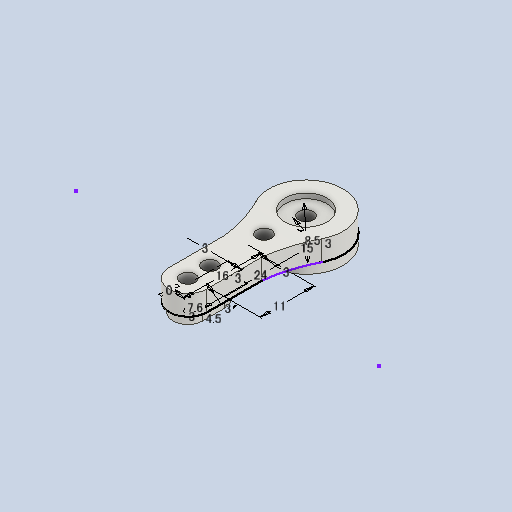
# Autodesk Inventor part: ServoMotor_Hone2
Saved by Autodesk Inventor 2022 (Build 260153000, 153)
## iProperties
Created: 2024-09-23
Part Number: ServoMotor_Hone2
Material: 鋼、高強度、低合金
Document SubType Name: Modeling
Designer: acbaf
Density: 7.85 g/cm^3
Appearance: 鋼
Author: acbaf
Autodesk Inventor part; units mm, degrees
ref_plane "YZ Plane" through (0, 0, 0) normal (1, 0, 0) x (0, 1, 0)
ref_plane "XZ Plane" through (0, 0, 0) normal (0, 1, 0) x (-1, 0, 0)
ref_plane "XY Plane" through (0, 0, 0) normal (0, 0, 1) x (1, 0, 0)
sketch "スケッチ1" plane through (0, 0, 0) normal (0, 1, 0) x (-1, 0, 0)
  circle A0 centre (0, 0) radius 7.5
  circle A1 centre (0, 0) radius 4.25
  circle A2 centre (0, 0) radius 1.5
  line L0 (0, 0) -> (0, 24)
  circle A3 centre (0, 24) radius 3.8
  line L1 (3.8, 24) -> (3.8, 12.8013)
  line L2 (-3.8, 24) -> (-3.8, 12.8013)
  circle A4 centre (0, 24) radius 1.5
  circle A5 centre (0, 19.5) radius 1.5
  circle A6 centre (0, 8.5) radius 1.5
  arc A7 (3.8, 12.8013) -> (6.6601, 3.4487) centre (30.7804, 15.9384) ccw
  arc A8 (-6.6601, 3.4487) -> (-3.8, 12.8013) centre (-30.7804, 15.9384) ccw
  line L3 (-3, 19.487) -> (3, 19.487)
  line L4 (3, 19.487) -> (3, 24.0195)
  line L5 (3, 24.0195) -> (-3, 24.0195)
  line L6 (-3, 24.0195) -> (-3, 19.487)
  circle A9 centre (0, 19.487) radius 3
  circle A10 centre (0, 24.0195) radius 3
  point P0 (3.8, 8)
  point P1 (-3.8, 8)
  point P2 (-6.6601, 3.4487)
  point P3 (3.8, 24)
  point P4 (-1.0476, 7.4265)
  point P5 (1.0476, 7.4265)
  dimension "d0" = 15
  dimension "d1" = 8.5
  dimension "d2" = 3
  dimension "d3" = 24
  dimension "d4" = 7.6
  dimension "d5" = 16
  dimension "d6" = 0
  dimension "d7" = 3
  dimension "d8" = 3
  dimension "d9" = 4.5
  dimension "d10" = 3
  dimension "d11" = 11
  dimension "d14" = 3
  dimension "d15" = 3
  constraints: 14 end point, 9 centre point, 5 coincident, 5 symmetric about line, 4 point on circle, 2 midpoint, 2 parallel, 2 point on line, 2 tangent, 2 vertical, 1 horizontal, 1 perpendicular, 8 other
  measures "d1" diameter of A1
  measures "d2" diameter of A2
  measures "d3" distance of L0.start L0.end
  measures "d4" diameter of A3
  measures "d5" distance of L1.start point (3.8, 8)
  measures "d6" vertical distance of L1.start A3.centre
  measures "d7" diameter of A4
  measures "d8" diameter of A5
  measures "d9" distance of A5.centre L0.end
  measures "d10" diameter of A6
  measures "d11" distance of A6.centre A5.centre
  measures "d14" distance between parallel lines of L0 L6
  measures "d15" distance between parallel lines of L4 L0
extrude "押し出し1" add sketch "スケッチ1" along normal blind 4 contours A0 A6 | A0 A6 L0 A9 L4 A3 L1 A7 | A8 L2 A3 L6 A9 L0 A6 A0 | A3 L4 A10 L6 | L4 A9 A3 | A3 A9 A10 L4 | A9 L3 A5 L0 | L0 A5 L3 A9 | L6 A10 A9 A3 | A3 A9 L6 | A9 L3 A5 A3 | A3 A5 L0 A10 A9 | A10 A9 L0 A4 L5 | L5 A4 A10 | A9 A3 A5 L3 | A9 A10 L0 A5 A3 | L5 A4 L0 A9 A10 | A10 L0 A9 | A9 L0 A10
extrude "押し出し2" add sketch "スケッチ1" against normal blind 2 contours L4 A9 A3 | A3 A9 A10 L4 | A9 L3 A5 L0 | L0 A5 L3 A9 | L6 A10 A9 A3 | A3 A9 L6 | A9 L3 A5 A3 | A3 A5 L0 A10 A9 | A10 A9 L0 A4 L5 | L5 A4 A10 | A9 A3 A5 L3 | A9 A10 L0 A5 A3 | L5 A4 L0 A9 A10 | A10 L0 A9 | A9 L0 A10
extrude "押し出し3" add sketch "スケッチ1" against normal blind 2 contours A0 A6
extrude "押し出し4" add sketch "スケッチ1" along normal blind 3 contours A1
